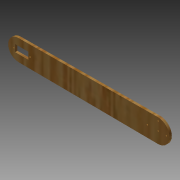
# Autodesk Inventor part: segment2a
Saved by Autodesk Inventor 2013 (Build 170138000, 138)
## iProperties
Created: 2014-10-09
Part Number: segment2a
Material: Generic
Document SubType Name: Modeling
Designer: Masta
Density: 1 g/cm^3
Author: Masta
Autodesk Inventor part; units mm, degrees
ref_plane "YZ Plane" through (0, 0, 0) normal (1, 0, 0) x (0, 1, 0)
ref_plane "XZ Plane" through (0, 0, 0) normal (0, 1, 0) x (-1, 0, 0)
ref_plane "XY Plane" through (0, 0, 0) normal (0, 0, 1) x (1, 0, 0)
sketch "Sketch1" plane through (0, 0, 0) normal (0, 1, 0) x (-1, 0, 0)
  arc A0 (0.1907, 19.9991) -> (0.1907, -19.9991) centre (0, 0) ccw
  arc A1 (0.1907, 19.9991) -> (240.1284, 17.9995) centre (953.4917, 100015.4551) ccw
  arc A2 (240.1284, -17.9995) -> (0.1907, -19.9991) centre (953.4917, -100015.4551) ccw
  arc A3 (240.1284, -17.9995) -> (240.1284, 17.9995) centre (240, 0) ccw
  line L0 (0, 0) -> (240, 0) construction
  line L1 (223, -6) -> (246, -6)
  line L2 (246, -6) -> (246, 6)
  line L3 (246, 6) -> (223, 6)
  line L4 (223, 6) -> (223, -6)
  line L5 (223, -6) -> (246, 6) construction
  line L6 (246, -6) -> (223, 6) construction
  line L7 (234.5, 0) -> (248.5, 0) construction
  line L8 (234.5, 0) -> (220.5, 0) construction
  line L9 (0, 0) -> (0, 15) construction
  line L10 (0, 0) -> (18.5, 0) construction
  line L11 (0, 0) -> (-14.5, 0) construction
  dimension "d2" = 40
  dimension "d10" = 100000
  dimension "d11" = 18
  dimension "d21" = 240
  dimension "d22" = 23
  dimension "d23" = 12
  dimension "d24" = 6
  dimension "d25" = 14
  dimension "d26" = 14
  dimension "d27" = 15
  dimension "d28" = 18.5
  dimension "d29" = 14.5
  constraints: 24 end point, 8 point on circle, 7 coincident, 4 centre point, 3 perpendicular, 3 point on line, 2 horizontal, 2 midpoint, 2 parallel, 2 tangent, 1 collinear, 1 other
  measures "d2" diameter of A0
  measures "d10" radius of A1
  measures "d11" radius of A3
  measures "d21" distance of L0.start L0.end
  measures "d22" distance of L3.end L2.end
  measures "d23" distance of L2.end L1.end
  measures "d24" distance from line of L0.end L2
  measures "d25" distance of L7.start L7.end
  measures "d26" distance of L7.start L8.end
  measures "d27" distance of L0.start L9.end
  measures "d28" distance of L0.start L10.end
  measures "d29" distance of L0.start L11.end
extrude "Extrusion1" add sketch "Sketch1" along normal blind 4
hole "Hole2" at (0, 0, 0) at (-248.5, 0, 0) at (-220.5, 0, 0) at (0, 0, 15) at (-18.5, 0, 0) at (14.5, 0, 0) direction (0, 1, 0) diameter 3 end through all
body "Solid1"
